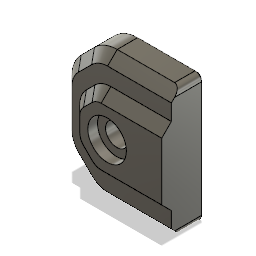
z_rail_stop_PARAMETRIC_x4 (Autodesk Fusion 360 design; units mm, degrees)
Autodesk Fusion 360 part; units mm, degrees
note: some values were not read from the file. Chosen so that the rebuilt part matches the saved one: which pieces of a blend or face edit are solid.
sketch "Sketch1" plane through (0, 0, 0) normal (0, 0, 1) x (1, 0, 0)
  line L0 (0, 0) -> (17, 0)
  line L1 (17, 0) -> (17, 20)
  line L2 (17, 20) -> (0, 20)
  line L3 (0, 20) -> (0, 0)
  circle A0 centre (8.5, 10) radius 3
  circle A1 centre (8.5, 10) radius 1.75
  line L4 (4.25, 14.5) -> (17, 14.5)
  line L5 (17, 14.5) -> (17, 5.5)
  line L6 (17, 5.5) -> (4.25, 5.5)
  line L7 (4.25, 5.5) -> (4.25, 14.5)
  line L8 (8.5, 10) -> (0, 10) construction
  line L9 (8.5, 10) -> (8.5, 20) construction
  dimension "d1" = 17
  dimension "d2" = 20
  dimension "d3" = 9
  dimension "d4" = 12.75
  dimension "d6" = 3.5
  dimension "d7" = 6
  measures "d1" distance of L0.start
  measures "d6" diameter of A1
  measures "d7" diameter of A0
extrude "Extrude1" add sketch "Sketch1" against normal blind 5 contours L0 L1 L2 L3 L4 L6 L7 | L1 L4 L5 L6 L7 | A0
extrude "Extrude2" add sketch "Sketch1" along normal blind 1.5 contours L1 L4 L5 L6 L7
chamfer "Chamfer1" distance 5 angle 45 2 edges at (0, 0, -2.5) (0, 20, -2.5)
chamfer "Chamfer2" distance 2.5 angle 45 2 edges at (4.25, 14.5, 0.75) (4.25, 5.5, 0.75)
fillet "Fillet1" radius 2 4 edges at (6.75, 5.5, 0.75) (4.25, 8, 0.75) (4.25, 12, 0.75) (6.75, 14.5, 0.75)
fillet "Fillet2" [suppressed]
fillet "Fillet3" radius 5 4 edges at (5, 20, -2.5) (0, 15, -2.5) (0, 5, -2.5) (5, 0, -2.5)
fillet "Fillet4" radius 1 2 edges at (17, 20, -2.5) (17, 0, -2.5)
fillet "Fillet5" [suppressed]
chamfer "Chamfer3" distance 0.3 angle 45 13 edges at (17, 10, -5) (16.7071, 19.7071, -5) (11.5355, 20, -5) (5.1577, 19.6194, -5) (2.5, 17.5, -5) (0.3806, 14.8423, -5) (0, 10, -5) (0.3806, 5.1577, -5) (2.5, 2.5, -5) (5.1577, 0.3806, -5) (11.5355, 0, -5) (16.7071, 0.2929, -5) (6.8684, 9.3672, -5)
chamfer "Chamfer4" distance 1.5 angle 45 18 edges at (11.5355, 20, 0) (5.1577, 19.6194, 0) (2.5, 17.5, 0) (0.3806, 14.8423, 0) (0, 10, 0) (0.3806, 5.1577, 0) (2.5, 2.5, 0) (5.1577, 0.3806, 0) (11.5355, 0, 0) (12.2892, 5.5, 0) (6.8131, 5.6522, 0) (5.5, 6.75, 0) (4.4022, 8.0631, 0) (4.25, 10, 0) (4.4022, 11.9369, 0) (5.5, 13.25, 0) (6.8131, 14.3478, 0) (12.2892, 14.5, 0)
equation "d1 = LENGTH"
equation "d4 = LENGTH * 0.75"
equation "LENGTH = 17 mm"
